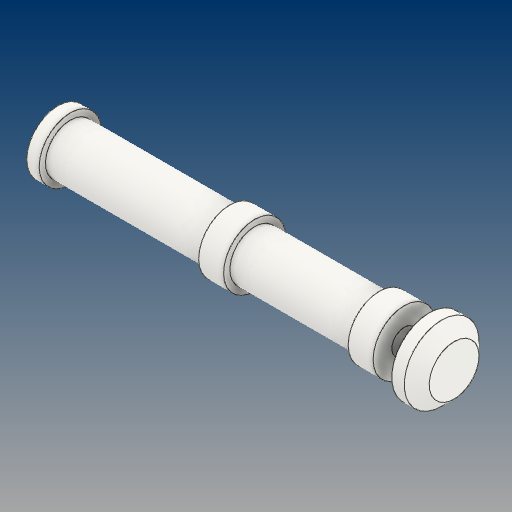
# Autodesk Inventor part: Shaft
Saved by Autodesk Inventor 2020 (Build 240168000, 168)
## iProperties
CustomPartVersion: 1
Created: 2020-08-26
Part Number: Shaft
Material: Steel
Document SubType Name: Modeling
Designer: alons
Density: 1 g/cm^3
Appearance: Steel
Length: 7.950 mm
Author: alons
Autodesk Inventor part; units mm, degrees
ref_plane "Start Plane" through (0, 0, 0) normal (1, 0, 0) x (0, 1, 0)
ref_plane "XZ Plane" through (0, 0, 0) normal (0, 1, 0) x (-1, 0, 0)
ref_plane "XY Plane" through (0, 0, 0) normal (0, 0, 1) x (1, 0, 0)
sketch "Main Sketch" plane through (0, 0, 0) normal (0, 0, 1) x (1, 0, 0)
  line L0 (0, 0) -> (7.95, 0)
  line L1 (0, 0) -> (0, 0.625)
  line L2 (3.45, 0.5) -> (3.45, 0.625)
  line L3 (0, 0.625) -> (0.25, 0.625)
  line L4 (3.95, 0.625) -> (3.95, 0.5)
  line L5 (3.45, 0.625) -> (3.95, 0.625)
  line L6 (7.45, 0.25) -> (7.45, 0.75)
  line L7 (6.95, 0.25) -> (7.45, 0.25)
  line L8 (7.95, 0.75) -> (7.95, 0)
  line L9 (7.45, 0.75) -> (7.95, 0.75)
  line L10 (0.25, 0.625) -> (0.25, 0.5)
  line L11 (0.25, 0.5) -> (3.45, 0.5)
  line L12 (3.7, 0.375) -> (6.2, 0.375)
  line L13 (6.2, 0.375) -> (6.2, 0.5)
  line L14 (6.7, 0.5) -> (6.7, 0.25)
  line L15 (6.2, 0.5) -> (6.7, 0.5)
  line L16 (3.95, 0.5) -> (6.45, 0.5)
  line L17 (6.45, 0.5) -> (6.45, 0.625)
  line L18 (6.95, 0.625) -> (6.95, 0.25)
  line L19 (6.45, 0.625) -> (6.95, 0.625)
  dimension "d3" = 1.25
  dimension "d6" = 1.25
  dimension "d7" = 0.5
  dimension "d10" = 1.5
  dimension "d15" = 1
  dimension "d22" = 0.75
  dimension "d23" = 1
  dimension "d24" = 1
  dimension "d25" = 1.25
  constraints: 40 end point, 10 vertical, 4 horizontal
  measures "d3" diameter of L3 L0
  measures "d6" diameter of L5 L0
  measures "d7" diameter of L7 L0
  measures "d10" diameter of L9 L0
  measures "d15" diameter of L11 L0
  measures "d22" diameter of L12 L0
  measures "d23" diameter of L15 L0
  measures "d24" diameter of L16 L0
  measures "d25" diameter of L19 L0
revolve "Revolution1" add sketch "Main Sketch" angle 360 about axis through (0, 0, 0) along (1, 0, 0)
chamfer "Chamfer3" [suppressed]
chamfer "Chamfer1" distance 0.25 angle 45 1 edges at (7.95, -0.75, 0) measured on face at (7.6167, 0.7476, -0.0603)
equation "\"Length\" = 7.95"
body "Solid1"
